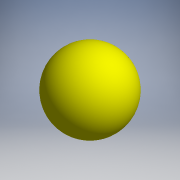
# Autodesk Inventor part: 30-62-38.1-18-ybrg1-61-9.525-46
Saved by Autodesk Inventor 2017.3 (Build 213256000, 256)
## iProperties
Part Number: 30-62-38.1-18-ybrg1-61-9.525-46
Material: Generic
Catalog Web Link: www.cadenas.de
Description: Ball for Y units-Y-bearings
Vendor: SKF
Document SubType Name: Modeling
Designer: partserver
Manufacturer: SKF
Mass: 0.452474 g
Surface Area: 2.85023 cm^2
Volume: 0.452474 cm^3
Density: 1 g/cm^3
Appearance: PSOLRGB-255-255-0
Category: PARTsolutions
Company: SKF
Title: 30-62-38.1-18-ybrg1-61-9.525-46
Author: Cadenas PARTsolutions
Comments: Y-bearings
PSOL_IDENT_0: {$CADENAS_DATA\23d-libs\skf\bearings_units_and_housings\bearing_units\ball_bearing_units\y-unit_acce
PSOL_IDENT_1: ssories\ball.prj},214 {VTYP=3D},{NB=30-62-38.1-18-ybrg1-61-9.525-46},{LINA=30-62-38.1-18-ybrg1-61-9.
PSOL_IDENT_2: 525-46},{NN=Ball for Y units},{DATE=20.08.2020 13:45:09},{GEOMDATE=29.07.2020 16:06:32},{VERSION=},{
PSOL_IDENT_3: LINEID=1580},{WBVAR=},{WBNUMERIC=}  {NB=30-62-38.1-18-ybrg1-61-9.525-46},{LINA=30-62-38.1-18-ybrg1-6
PSOL_IDENT_4: 1-9.525-46},{KT=DUMMY},{DD=30.0000},{D=62},{B=38.100},{C=18.000},{PITCH=46.000},{DW=9.525},{FO=IEC_B
PSOL_IDENT_5: BY_006},{DESIGN=ybrg1},{X=0},{PN=61}
NB: 30-62-38.1-18-ybrg1-61-9.525-46
NN: Ball for Y units
NT: Y-bearings
NBSYN: $DD.-$D.-$B.-$C.-$DESIGN.-$PN.-$DW.-$PITCH.
LINA: 30-62-38.1-18-ybrg1-61-9.525-46
CATALOG: SKF
DD: 30
D: 62
B: 38.1
C: 18
PITCH: 46
DW: 9.525
FO: IEC_BBY_006
DESIGN: ybrg1
SUPPLIER: SKF
ARTICLENO: 30-62-38.1-18-ybrg1-61-9.525-46
BOMINFO: 30-62-38.1-18-ybrg1-61-9.525-46
CREATOR: CADENAS GmbH
Autodesk Inventor part; units mm, degrees
sketch "Sketch_1" plane through (0, 0, 0) normal (0, 0, 1) x (1, 0, 0)
  line L0 (4.7625, 23) -> (-4.7625, 23)
  arc A0 (4.7625, 23) -> (-4.7625, 23) centre (0, 23) ccw
  line L1 (4.7625, 23) -> (-4.7625, 23)
  constraints: 4 end point, 2 point on circle, 1 centre point
revolve "Revolution1" add sketch "Sketch_1" angle 360 about axis through (4.7625, 23, 0) along (1, 0, 0)
ref_plane "ball_XY" through (0, 23, 0) normal (1, 0, 0) x (0, 0, -1)
ref_plane "ball_YZ" through (0, 23, 0) normal (0, 0, -1) x (0, 1, 0)
ref_plane "ball_ZX" through (0, 23, 0) normal (0, 1, 0) x (1, 0, 0)
body "Solid1"
